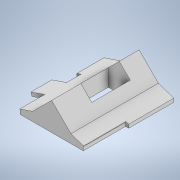
# Autodesk Inventor part: 12-12-PartOfHouseRoof
Saved by Autodesk Inventor 2022 (Build 260153070, 153G)
## iProperties
Created: 2021-07-13
Part Number: 12-12-PartOfHouseRoof
Material: Generic
Document SubType Name: Modeling
Designer: robst
Density: 1 g/cm^3
Appearance: Default
Author: robst
Autodesk Inventor part; units mm, degrees
ref_plane "YZ Plane" through (0, 0, 0) normal (1, 0, 0) x (0, 1, 0)
ref_plane "XY Plane" through (0, 0, 0) normal (0, 0, 1) x (1, 0, 0)
sketch "Sketch1" plane through (0, 0, 0) normal (0, 0, 1) x (1, 0, 0)
  line L0 (0, 0) -> (-6129.9427, 0)
  line L1 (-6129.9427, 0) -> (-3322.6948, 935.7521)
  line L2 (-3322.6948, 935.7521) -> (-1557.9427, 935.7521) construction
  line L3 (-3322.6948, 935.7521) -> (0, 4258.4469)
  line L4 (0, 4258.4469) -> (0, 0) construction
  line L5 (0, 4258.4469) -> (3358.6158, 899.8311)
  line L6 (3358.6158, 899.8311) -> (0, 899.8311) construction
  line L7 (3358.6158, 899.8311) -> (6058.1009, 0)
  line L8 (6058.1009, 0) -> (0, 0)
  dimension "d1" = 18.435
  dimension "d2" = 2959.1
  dimension "d4" = 45
  dimension "d6" = 4699
  dimension "d7" = 45
  dimension "d8" = 4749.8
  dimension "d9" = 18.435
  dimension "d10" = 2845.508
  constraints: 18 end point, 3 horizontal, 1 perpendicular, 1 point on line, 1 vertical
  measures "d1" angle of L1 L0
  measures "d2" distance of L0.end L1.end
  measures "d4" angle of L3 L2
  measures "d6" distance of L1.end L3.end
  measures "d7" angle of L5 L6
  measures "d8" distance of L3.end L5.end
  measures "d9" angle of L7 L8
  measures "d10" distance of L5.end L7.end
extrude "Extrusion1" add sketch "Sketch1" along normal blind 15240
sketch "Sketch2" plane through (3358.6158, 899.8311, 15240) normal (0.3162286, 0.948683, 0) x (0.948683, -0.3162286, 0)
  line L0 (2845.5081, 0) -> (0, 0) projected
  line L1 (2845.5081, 0) -> (2324.1, 0)
  line L2 (2324.1, 0) -> (2324.1, 7366)
  line L3 (2324.1, 7366) -> (2845.5081, 7366)
  line L4 (2845.5081, 7366) -> (2845.5081, 0)
  line L5 (2845.5081, 15240) -> (0, 15240) projected
  line L6 (0, 15240) -> (0, 0) projected
  point P0 (-2901.7094, 15240)
  point P1 (2324.1, 0)
  dimension "d13" = 7874
  dimension "d14" = 2324.1
  constraints: 8 end point, 2 parallel, 1 horizontal, 1 perpendicular
  measures "d13" distance between parallel lines of L3 L5
  measures "d14" distance between parallel lines of L2 L6
extrude "Extrusion2" cut sketch "Sketch2" against normal through all
sketch "Sketch3" plane through (-6129.9427, 0, 15240) normal (-0.3162286, 0.948683, 0) x (0.948683, 0.3162286, 0)
  line L0 (0, 0) -> (622.3, 0)
  line L1 (622.3, 0) -> (622.3, 4318)
  line L2 (622.3, 4318) -> (0, 4318)
  line L3 (0, 4318) -> (0, 0)
  line L4 (2959.1, 15240) -> (2959.1, 0) projected
  point P0 (5815.3725, 15240)
  dimension "d17" = 2336.8
  dimension "d18" = 4318
  constraints: 8 end point, 2 parallel, 1 horizontal, 1 perpendicular
  measures "d17" distance between parallel lines of L1 L4
  measures "d18" distance between parallel lines of L0 L2
extrude "Extrusion3" cut sketch "Sketch3" against normal through all
sketch "Sketch4" plane through (-3322.6948, 935.7521, 15240) normal (-0.3162286, 0.948683, 0) x (0.948683, 0.3162286, 0)
  line L0 (-2959.1, 15240) -> (-2959.1, 4318) projected
  line L1 (-2959.1, 10490.2) -> (-2184.4, 10490.2)
  line L2 (-2184.4, 10490.2) -> (-2184.4, 7975.6)
  line L3 (-2184.4, 7975.6) -> (-2959.1, 7975.6)
  line L4 (-2959.1, 7975.6) -> (-2959.1, 10490.2)
  line L5 (0, 15240) -> (-2959.1, 15240) projected
  line L6 (0, 15240) -> (0, 0) projected
  line L7 (-2959.1, 4318) -> (-2336.8, 4318) projected
  point P0 (2856.2725, 15240)
  point P1 (-2959.1, 7975.6)
  dimension "d22" = 4749.8
  dimension "d23" = 2184.4
  dimension "d24" = 3657.6
  constraints: 8 end point, 2 parallel, 1 horizontal, 1 perpendicular, 1 point on line
  measures "d22" distance between parallel lines of L1 L5
  measures "d23" distance between parallel lines of L2 L6
  measures "d24" distance between parallel lines of L3 L7
extrude "Extrusion4" cut sketch "Sketch4" against normal through all
sketch "Sketch5" plane through (-6129.9427, 0, 0) normal (0, -1, 0) x (1, 0, 0)
  line L0 (655.962, 15240) -> (11638.4311, 15240) projected
  line L1 (655.962, 15240) -> (11638.4311, 15240)
  line L2 (11693.3927, 7874) -> (11638.4311, 7874) projected
  line L3 (11638.4311, 15240) -> (11638.4311, 7874)
  line L4 (11638.4311, 7874) -> (12188.0436, 7874)
  line L5 (12188.0436, 0) -> (9488.5585, 0) projected
  line L6 (12188.0436, 7874) -> (12188.0436, 0)
  line L7 (2807.2479, 0) -> (0, 0) projected
  line L8 (12188.0436, 0) -> (0, 0)
  line L9 (0, 0) -> (0, 4749.8) projected
  line L10 (0, 0) -> (0, 4749.8)
  line L11 (816.6057, 4749.8) -> (0, 4749.8) projected
  line L12 (0, 4749.8) -> (816.6057, 4749.8)
  line L13 (734.9447, 7264.4) -> (816.6057, 7264.4) projected
  line L14 (816.6057, 4749.8) -> (816.6057, 7264.4)
  line L15 (734.9447, 7264.4) -> (0, 7264.4) projected
  line L16 (816.6057, 7264.4) -> (0, 7264.4)
  line L17 (0, 7264.4) -> (0, 10922) projected
  line L18 (0, 7264.4) -> (0, 10922)
  line L19 (655.962, 15240) -> (655.962, 10922) projected
  line L20 (0, 10922) -> (655.962, 10922)
  line L21 (655.962, 10922) -> (655.962, 15240)
  point P0 (6129.9427, 0)
  constraints: 24 end point, 9 perpendicular, 3 collinear
extrude "Extrusion5" add sketch "Sketch5" along normal blind 609.6
sketch "Sketch6" plane through (-3322.6948, 935.7521, 15240) normal (-0.3162286, 0.948683, 0) x (0.948683, 0.3162286, 0)
  line L0 (-2184.4, 7975.6) -> (-2959.1, 7975.6) projected
  line L1 (-2959.1, 7975.6) -> (-4864.1, 7975.6)
  line L2 (-4864.1, 7975.6) -> (-4864.1, 4318)
  line L3 (-4864.1, 4318) -> (-2959.1, 4318)
  line L4 (-2959.1, 4318) -> (-2959.1, 7975.6)
  point P0 (2856.2725, 15240)
  dimension "d29" = 1905
  constraints: 8 end point, 2 parallel, 1 horizontal, 1 perpendicular
  measures "d29" distance of L3.end L2.end
extrude "Extrusion6" add sketch "Sketch6" against normal blind 609.6
ref_plane "Work Plane1" through (0, 4258.4469, 15240) normal (0, 1, 0) x (-1, 0, 0)
sketch "Sketch7" plane through (0, 4258.4469, 15240) normal (0, 1, 0) x (-1, 0, 0)
  line L0 (1905, -5080) -> (-1905, -5080)
  line L1 (-1905, -5080) -> (-1905, -11785.6)
  line L2 (-1905, -11785.6) -> (1905, -11785.6)
  line L3 (1905, -11785.6) -> (1905, -5080)
  line L4 (0, -15240) -> (0, 0) projected
  line L5 (1905, -5080) -> (-1905, -11785.6) construction
  line L6 (-1905, -5080) -> (1905, -11785.6) construction
  point P0 (0, -8432.8)
  dimension "d32" = 5080
  dimension "d33" = 6705.6
  dimension "d34" = 3810
  constraints: 12 end point, 2 midpoint, 2 parallel, 2 perpendicular, 1 point on line
  measures "d32" distance from line of L0 L4.end
  measures "d33" distance of L0.end L1.end
  measures "d34" distance of L1.end L2.end
extrude "Extrusion7" cut sketch "Sketch7" against normal through all
equation "\"d1\" = pitch_4_12"
equation "\"d4\" = pitch_12_12"
equation "\"d7\" = pitch_12_12"
equation "\"d9\" = pitch_4_12"
equation "\"pitch_4_12\" = 18.435deg"
equation "\"pitch_12_12\" = 45deg"
body "Solid1"
